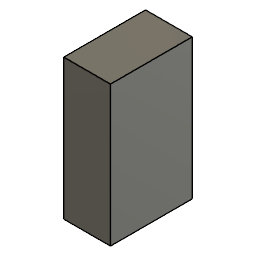
box_yz_run01 (Autodesk Fusion 360 design; units mm, degrees)
Autodesk Fusion 360 part; units mm, degrees
sketch "草图1" plane through (0, 0, 0) normal (1, 0, 0) x (0, 0, -1)
  line L0 (0, 0) -> (0, 48)
  line L1 (0, 48) -> (-28, 48)
  line L2 (-28, 48) -> (-28, 0)
  line L3 (-28, 0) -> (0, 0)
extrude "拉伸1" add sketch "草图1" along normal blind 16
